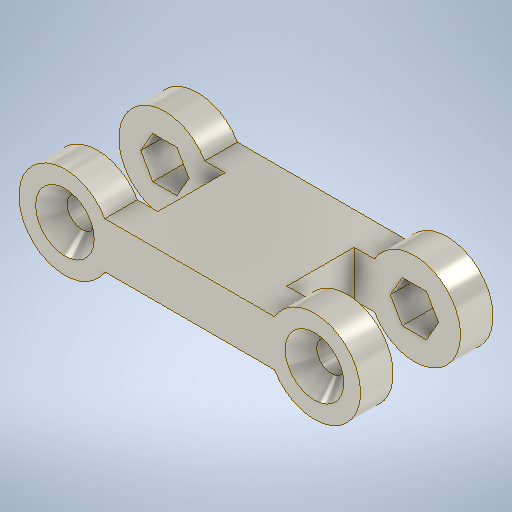
# Autodesk Inventor part: Barra1_0001_001
Saved by Autodesk Inventor 2025.2 (Build 292293000, 293)
## iProperties
Created: 2025-05-22
Part Number: Barra1_0001_001
Material: Titânio
Document SubType Name: Modeling
Designer: Gustavo Sousa
Density: 4.51 g/cm^3
Appearance: Titânio
Author: Gustavo Sousa
Autodesk Inventor part; units mm, degrees
ref_plane "YZ Plane" through (0, 0, 0) normal (1, 0, 0) x (0, 1, 0)
ref_plane "XZ Plane" through (0, 0, 0) normal (0, 1, 0) x (-1, 0, 0)
ref_plane "XY Plane" through (0, 0, 0) normal (0, 0, 1) x (1, 0, 0)
sketch "Esboço1" plane through (0, 0, 0) normal (0, 0, 1) x (1, 0, 0)
  line L0 (-10.1444, 2.75) -> (10.1444, 2.75)
  line L1 (-10.1444, -2.75) -> (10.1444, -2.75)
  circle A0 centre (-14.9075, 0) radius 5.5
  circle A1 centre (14.9075, 0) radius 5.5
  circle A2 centre (-14.9075, 0) radius 3.5
  circle A3 centre (14.9075, 0) radius 3.5
  point P0 (0, 0)
  point P1 (0, 2.75)
  point P2 (0, -2.75)
  dimension "d7" = 11
  dimension "d5" = 2.75
  dimension "d6" = 2.75
  dimension "d9" = 14.9075
  dimension "d11" = 29.815
  dimension "d12" = 7
  dimension "d13" = 7
  constraints: 4 end point, 3 centre point, 2 coincident, 2 horizontal, 2 horizontal alignment, 2 midpoint, 2 vertical alignment, 1 parallel, 4 other
  measures "d5" distance of point (0, 0) point (0, 2.75)
  measures "d6" distance of point (0, 0) point (0, -2.75)
  measures "d9" distance of point (0, 0) point (-14.908, 0)
  measures "d11" distance of point (-14.908, 0) A1.centre
  measures "d12" diameter of A2
  measures "d13" diameter of A3
extrude "Extrusão1" add sketch "Esboço1" along normal mid plane 3.9 contours L0 A1 L1 A0 | A0 | A1 | A2 | A3
sketch "Esboço2" plane through (0, 0, -1.95) normal (0, 0, -1) x (-1, 0, 0)
  line L0 (-7.7154, -2.75) -> (7.7154, -2.75)
  line L1 (7.7154, -2.75) -> (7.7154, 2.75)
  line L2 (7.7154, 2.75) -> (-7.7154, 2.75)
  line L3 (-7.7154, 2.75) -> (-7.7154, -2.75)
  line L4 (-7.7154, -2.75) -> (7.7154, 2.75) construction
  line L5 (7.7154, -2.75) -> (-7.7154, 2.75) construction
  line L6 (10.1444, 2.75) -> (-10.1444, 2.75) projected
  line L7 (-10.1444, -2.75) -> (10.1444, -2.75) projected
  point P0 (0, 0)
  point P1 (0, 2.75)
  point P2 (0, -2.75)
  point P3 (7.7154, 0)
  point P4 (0, 2.75)
  dimension "d21" = 15.4307
  constraints: 12 end point, 8 midpoint, 1 horizontal, 1 horizontal alignment, 1 parallel, 1 perpendicular, 1 vertical alignment
  measures "d21" distance of L1.end L2.end
extrude "Extrusão2" add sketch "Esboço2" along normal blind 8.04
sketch "Esboço3" plane through (0, 0, 1.95) normal (0, 0, 1) x (1, 0, 0)
  arc A0 (10.1444, -2.75) -> (10.1444, 2.75) centre (14.9075, 0) ccw projected
  point P0 (0, 0)
  constraints: 1 coincident
hole "Furo1" at (14.9075, 0, 1.95) direction (0, 0, -1) diameter 3.5 end through all countersink diameter 7 countersink angle 82
sketch "Esboço4" plane through (0, 0, 1.95) normal (0, 0, 1) x (1, 0, 0)
  arc A0 (-10.1444, 2.75) -> (-10.1444, -2.75) centre (-14.9075, 0) ccw projected
  point P0 (0, 0)
  constraints: 1 coincident
hole "Furo2" at (-14.9075, 0, 1.95) direction (0, 0, -1) diameter 3.5 end through all countersink diameter 7 countersink angle 82
sketch "Esboço5" plane through (0, 0, -9.99) normal (0, 0, -1) x (-1, 0, 0)
  arc A0 (-10.1444, 2.75) -> (-10.1444, -2.75) centre (-14.9075, 0) ccw projected
  circle A1 centre (-14.9075, 0) radius 5.5
  arc A2 (10.1444, -2.75) -> (10.1444, 2.75) centre (14.9075, 0) ccw projected
  circle A3 centre (14.9075, 0) radius 5.5
  line L0 (-10.1444, 2.75) -> (10.1444, 2.75)
  line L1 (-10.1444, -2.75) -> (10.1444, -2.75)
  line L2 (-13.4641, 2.5) -> (-12.0207, 0)
  line L3 (-12.0207, 0) -> (-13.4641, -2.5)
  line L4 (-13.4641, -2.5) -> (-16.3509, -2.5)
  line L5 (-16.3509, -2.5) -> (-17.7943, 0)
  line L6 (-17.7943, 0) -> (-16.3509, 2.5)
  line L7 (-16.3509, 2.5) -> (-13.4641, 2.5)
  line L8 (16.3509, 2.5) -> (17.7943, 0)
  line L9 (17.7943, 0) -> (16.3509, -2.5)
  line L10 (16.3509, -2.5) -> (13.4641, -2.5)
  line L11 (13.4641, -2.5) -> (12.0207, 0)
  line L12 (12.0207, 0) -> (13.4641, 2.5)
  line L13 (13.4641, 2.5) -> (16.3509, 2.5)
  point P0 (0, 0)
  point P1 (-14.9075, 2.5)
  point P2 (14.9075, 2.5)
  dimension "d37" = 11
  dimension "d38" = 3
  dimension "d39" = 3
  constraints: 28 end point, 4 coincident, 2 horizontal alignment, 2 midpoint, 2 vertical alignment, 1 centre point, 1 horizontal, 29 other
  measures "d37" diameter of A1
  measures "d38" distance edge to line of A0 L7
extrude "Extrusão3" add sketch "Esboço5" along normal blind 3.9
equation "\"d6\" = d5"
